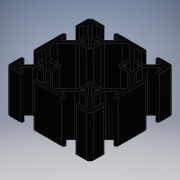
# Autodesk Inventor part: 2020-S-BLACK-FB
Saved by Autodesk Inventor 2017 SP1 (Build 210196100, 196)
## iProperties
Created: 2016-09-13
Part Number: 2020-S-BLACK-FB
Material: 6105-T5
Description: 40 S SHORT SINGLE UNIBEARING ASSEMBLY ON 40-4040 X 75mm
Document SubType Name: Modeling
Designer: BRALEF
Density: 1 g/cm^3
Appearance: BLACK ANODIZED
MATERIAL: 6061-T6
PART PRICE: 44.65
Author: BRALEF
Autodesk Inventor part; units mm, degrees
ref_plane "YZ Plane" through (0, 0, 0) normal (1, 0, 0) x (0, 1, 0)
ref_plane "XZ Plane" through (0, 0, 0) normal (0, 1, 0) x (-1, 0, 0)
ref_plane "XY Plane" through (0, 0, 0) normal (0, 0, 1) x (1, 0, 0)
sketch "Sketch1" plane through (0, 0, 0) normal (0, 1, 0) x (-1, 0, 0)
  arc A0 (-4.5172, 2.0392) -> (-5.1644, 3.6017) centre (-6.727, 2.0392) ccw
  line L0 (-10.6413, 9.0787) -> (-5.1644, 3.6017)
  arc A1 (-10.6413, 9.0787) -> (-14.7587, 9.0787) centre (-12.7, 7.02) ccw
  line L1 (-20.2356, 3.6017) -> (-14.7587, 9.0787)
  arc A2 (-20.2356, 3.6017) -> (-20.8828, 2.0392) centre (-18.673, 2.0392) ccw
  line L2 (-20.8828, -2.3074) -> (-20.8828, 2.0392)
  arc A3 (-23.0926, -4.5172) -> (-20.8828, -2.3074) centre (-23.0926, -2.3074) ccw
  line L3 (-27.4392, -4.5172) -> (-23.0926, -4.5172)
  arc A4 (-27.4392, -4.5172) -> (-29.0017, -5.1644) centre (-27.4392, -6.727) ccw
  line L4 (-34.4787, -10.6413) -> (-29.0017, -5.1644)
  arc A5 (-34.4787, -10.6413) -> (-34.4787, -14.7587) centre (-32.42, -12.7) ccw
  line L5 (-29.0017, -20.2356) -> (-34.4787, -14.7587)
  arc A6 (-29.0017, -20.2356) -> (-27.4392, -20.8828) centre (-27.4392, -18.673) ccw
  line L6 (-23.0926, -20.8828) -> (-27.4392, -20.8828)
  arc A7 (-20.8828, -23.0926) -> (-23.0926, -20.8828) centre (-23.0926, -23.0926) ccw
  line L7 (-20.8828, -27.4392) -> (-20.8828, -23.0926)
  arc A8 (-20.8828, -27.4392) -> (-20.2356, -29.0017) centre (-18.673, -27.4392) ccw
  line L8 (-14.7587, -34.4787) -> (-20.2356, -29.0017)
  arc A9 (-14.7587, -34.4787) -> (-10.6413, -34.4787) centre (-12.7, -32.42) ccw
  line L9 (-5.1644, -29.0017) -> (-10.6413, -34.4787)
  arc A10 (-5.1644, -29.0017) -> (-4.5172, -27.4392) centre (-6.727, -27.4392) ccw
  line L10 (-4.5172, -23.0926) -> (-4.5172, -27.4392)
  arc A11 (-2.3074, -20.8828) -> (-4.5172, -23.0926) centre (-2.3074, -23.0926) ccw
  line L11 (2.0392, -20.8828) -> (-2.3074, -20.8828)
  arc A12 (2.0392, -20.8828) -> (3.6017, -20.2356) centre (2.0392, -18.673) ccw
  line L12 (9.0787, -14.7587) -> (3.6017, -20.2356)
  arc A13 (9.0787, -14.7587) -> (9.0787, -10.6413) centre (7.02, -12.7) ccw
  line L13 (3.6017, -5.1644) -> (9.0787, -10.6413)
  arc A14 (3.6017, -5.1644) -> (2.0392, -4.5172) centre (2.0392, -6.727) ccw
  line L14 (-2.3074, -4.5172) -> (2.0392, -4.5172)
  arc A15 (-4.5172, -2.3074) -> (-2.3074, -4.5172) centre (-2.3074, -2.3074) ccw
  line L15 (-4.5172, 2.0392) -> (-4.5172, -2.3074)
  arc A16 (-2.8605, -1.9692) -> (-1.9692, -2.8605) centre (-2.4696, -2.4696) ccw
  line L16 (-1.3405, -2.2319) -> (-1.9692, -2.8605)
  arc A17 (-1.3405, -2.2319) -> (1.3405, -2.2319) centre (0, 0) ccw
  line L17 (1.9692, -2.8605) -> (1.3405, -2.2319)
  arc A18 (1.9692, -2.8605) -> (2.8605, -1.9692) centre (2.4696, -2.4696) ccw
  line L18 (2.2319, -1.3405) -> (2.8605, -1.9692)
  arc A19 (2.2319, -1.3405) -> (2.2319, 1.3405) centre (0, 0) ccw
  line L19 (2.8605, 1.9692) -> (2.2319, 1.3405)
  arc A20 (2.8605, 1.9692) -> (1.9692, 2.8605) centre (2.4696, 2.4696) ccw
  line L20 (1.3405, 2.2319) -> (1.9692, 2.8605)
  arc A21 (1.3405, 2.2319) -> (-1.3405, 2.2319) centre (0, 0) ccw
  line L21 (-1.9692, 2.8605) -> (-1.3405, 2.2319)
  arc A22 (-1.9692, 2.8605) -> (-2.8605, 1.9692) centre (-2.4696, 2.4696) ccw
  line L22 (-2.2319, 1.3405) -> (-2.8605, 1.9692)
  arc A23 (-2.2319, 1.3405) -> (-2.2319, -1.3405) centre (0, 0) ccw
  line L23 (-2.8605, -1.9692) -> (-2.2319, -1.3405)
  arc A24 (-28.2605, -1.9692) -> (-27.3692, -2.8605) centre (-27.8696, -2.4696) ccw
  line L24 (-26.7405, -2.2319) -> (-27.3692, -2.8605)
  arc A25 (-26.7405, -2.2319) -> (-24.0595, -2.2319) centre (-25.4, 0) ccw
  line L25 (-23.4308, -2.8605) -> (-24.0595, -2.2319)
  arc A26 (-23.4308, -2.8605) -> (-22.5395, -1.9692) centre (-22.9304, -2.4696) ccw
  line L26 (-23.1681, -1.3405) -> (-22.5395, -1.9692)
  arc A27 (-23.1681, -1.3405) -> (-23.1681, 1.3405) centre (-25.4, 0) ccw
  line L27 (-22.5395, 1.9692) -> (-23.1681, 1.3405)
  arc A28 (-22.5395, 1.9692) -> (-23.4308, 2.8605) centre (-22.9304, 2.4696) ccw
  line L28 (-24.0595, 2.2319) -> (-23.4308, 2.8605)
  arc A29 (-24.0595, 2.2319) -> (-26.7405, 2.2319) centre (-25.4, 0) ccw
  line L29 (-27.3692, 2.8605) -> (-26.7405, 2.2319)
  arc A30 (-27.3692, 2.8605) -> (-28.2605, 1.9692) centre (-27.8696, 2.4696) ccw
  line L30 (-27.6319, 1.3405) -> (-28.2605, 1.9692)
  arc A31 (-27.6319, 1.3405) -> (-27.6319, -1.3405) centre (-25.4, 0) ccw
  line L31 (-28.2605, -1.9692) -> (-27.6319, -1.3405)
  arc A32 (1.3405, -23.1681) -> (-1.3405, -23.1681) centre (0, -25.4) ccw
  line L32 (-1.9692, -22.5395) -> (-1.3405, -23.1681)
  arc A33 (-1.9692, -22.5395) -> (-2.8605, -23.4308) centre (-2.4696, -22.9304) ccw
  line L33 (-2.2319, -24.0595) -> (-2.8605, -23.4308)
  arc A34 (-2.2319, -24.0595) -> (-2.2319, -26.7405) centre (0, -25.4) ccw
  line L34 (-2.8605, -27.3692) -> (-2.2319, -26.7405)
  arc A35 (-2.8605, -27.3692) -> (-1.9692, -28.2605) centre (-2.4696, -27.8696) ccw
  line L35 (-1.3405, -27.6319) -> (-1.9692, -28.2605)
  arc A36 (-1.3405, -27.6319) -> (1.3405, -27.6319) centre (0, -25.4) ccw
  line L36 (1.9692, -28.2605) -> (1.3405, -27.6319)
  arc A37 (1.9692, -28.2605) -> (2.8605, -27.3692) centre (2.4696, -27.8696) ccw
  line L37 (2.2319, -26.7405) -> (2.8605, -27.3692)
  arc A38 (2.2319, -26.7405) -> (2.2319, -24.0595) centre (0, -25.4) ccw
  line L38 (2.8605, -23.4308) -> (2.2319, -24.0595)
  arc A39 (2.8605, -23.4308) -> (1.9692, -22.5395) centre (2.4696, -22.9304) ccw
  line L39 (1.3405, -23.1681) -> (1.9692, -22.5395)
  arc A40 (-28.2605, -27.3692) -> (-27.3692, -28.2605) centre (-27.8696, -27.8696) ccw
  line L40 (-26.7405, -27.6319) -> (-27.3692, -28.2605)
  arc A41 (-26.7405, -27.6319) -> (-24.0595, -27.6319) centre (-25.4, -25.4) ccw
  line L41 (-23.4308, -28.2605) -> (-24.0595, -27.6319)
  arc A42 (-23.4308, -28.2605) -> (-22.5395, -27.3692) centre (-22.9304, -27.8696) ccw
  line L42 (-23.1681, -26.7405) -> (-22.5395, -27.3692)
  arc A43 (-23.1681, -26.7405) -> (-23.1681, -24.0595) centre (-25.4, -25.4) ccw
  line L43 (-22.5395, -23.4308) -> (-23.1681, -24.0595)
  arc A44 (-22.5395, -23.4308) -> (-23.4308, -22.5395) centre (-22.9304, -22.9304) ccw
  line L44 (-24.0595, -23.1681) -> (-23.4308, -22.5395)
  arc A45 (-24.0595, -23.1681) -> (-26.7405, -23.1681) centre (-25.4, -25.4) ccw
  line L45 (-27.3692, -22.5395) -> (-26.7405, -23.1681)
  arc A46 (-27.3692, -22.5395) -> (-28.2605, -23.4308) centre (-27.8696, -22.9304) ccw
  line L46 (-27.6319, -24.0595) -> (-28.2605, -23.4308)
  arc A47 (-27.6319, -24.0595) -> (-27.6319, -26.7405) centre (-25.4, -25.4) ccw
  line L47 (-28.2605, -27.3692) -> (-27.6319, -26.7405)
  arc A48 (12.7, -29.7561) -> (10.4902, -29.7561) centre (11.5951, -29.7561) ccw
  line L48 (12.7, -29.7561) -> (12.7, -35.9918)
  arc A49 (10.5918, -38.1) -> (12.7, -35.9918) centre (10.5918, -35.9918) ccw
  line L49 (10.5918, -38.1) -> (4.3561, -38.1)
  arc A50 (4.3561, -35.8902) -> (4.3561, -38.1) centre (4.3561, -36.9951) ccw
  line L50 (4.3561, -35.8902) -> (6.4749, -35.8902)
  arc A51 (6.4749, -35.8902) -> (7.1933, -34.1558) centre (6.4749, -34.8742) ccw
  line L51 (7.1933, -34.1558) -> (3.8846, -30.8471)
  arc A52 (3.8846, -30.8471) -> (1.6396, -29.9172) centre (1.6396, -33.0922) ccw
  line L52 (1.6396, -29.9172) -> (-1.6396, -29.9172)
  arc A53 (-1.6396, -29.9172) -> (-3.8846, -30.8471) centre (-1.6396, -33.0922) ccw
  line L53 (-3.8846, -30.8471) -> (-7.1933, -34.1558)
  arc A54 (-7.1933, -34.1558) -> (-6.4749, -35.8902) centre (-6.4749, -34.8742) ccw
  line L54 (-6.4749, -35.8902) -> (-4.3561, -35.8902)
  arc A55 (-4.3561, -38.1) -> (-4.3561, -35.8902) centre (-4.3561, -36.9951) ccw
  line L55 (-4.3561, -38.1) -> (-21.0439, -38.1)
  arc A56 (-21.0439, -35.8902) -> (-21.0439, -38.1) centre (-21.0439, -36.9951) ccw
  line L56 (-21.0439, -35.8902) -> (-18.9251, -35.8902)
  arc A57 (-18.9251, -35.8902) -> (-18.2067, -34.1558) centre (-18.9251, -34.8742) ccw
  line L57 (-18.2067, -34.1558) -> (-21.5154, -30.8471)
  arc A58 (-21.5154, -30.8471) -> (-23.7604, -29.9172) centre (-23.7604, -33.0922) ccw
  line L58 (-23.7604, -29.9172) -> (-27.0396, -29.9172)
  arc A59 (-27.0396, -29.9172) -> (-29.2846, -30.8471) centre (-27.0396, -33.0922) ccw
  line L59 (-29.2846, -30.8471) -> (-32.5933, -34.1558)
  arc A60 (-32.5933, -34.1558) -> (-31.8749, -35.8902) centre (-31.8749, -34.8742) ccw
  line L60 (-31.8749, -35.8902) -> (-29.7561, -35.8902)
  arc A61 (-29.7561, -38.1) -> (-29.7561, -35.8902) centre (-29.7561, -36.9951) ccw
  line L61 (-29.7561, -38.1) -> (-35.9918, -38.1)
  arc A62 (-38.1, -35.9918) -> (-35.9918, -38.1) centre (-35.9918, -35.9918) ccw
  line L62 (-38.1, -35.9918) -> (-38.1, -29.7561)
  arc A63 (-35.8902, -29.7561) -> (-38.1, -29.7561) centre (-36.9951, -29.7561) ccw
  line L63 (-35.8902, -29.7561) -> (-35.8902, -31.8749)
  arc A64 (-35.8902, -31.8749) -> (-34.1558, -32.5933) centre (-34.8742, -31.8749) ccw
  line L64 (-34.1558, -32.5933) -> (-30.8471, -29.2846)
  arc A65 (-30.8471, -29.2846) -> (-29.9172, -27.0396) centre (-33.0922, -27.0396) ccw
  line L65 (-29.9172, -27.0396) -> (-29.9172, -23.7604)
  arc A66 (-29.9172, -23.7604) -> (-30.8471, -21.5154) centre (-33.0922, -23.7604) ccw
  line L66 (-30.8471, -21.5154) -> (-34.1558, -18.2067)
  arc A67 (-34.1558, -18.2067) -> (-35.8902, -18.9251) centre (-34.8742, -18.9251) ccw
  line L67 (-35.8902, -18.9251) -> (-35.8902, -21.0439)
  arc A68 (-38.1, -21.0439) -> (-35.8902, -21.0439) centre (-36.9951, -21.0439) ccw
  line L68 (-38.1, -21.0439) -> (-38.1, -4.3561)
  arc A69 (-35.8902, -4.3561) -> (-38.1, -4.3561) centre (-36.9951, -4.3561) ccw
  line L69 (-35.8902, -4.3561) -> (-35.8902, -6.4749)
  arc A70 (-35.8902, -6.4749) -> (-34.1558, -7.1933) centre (-34.8742, -6.4749) ccw
  line L70 (-34.1558, -7.1933) -> (-30.8471, -3.8846)
  arc A71 (-30.8471, -3.8846) -> (-29.9172, -1.6396) centre (-33.0922, -1.6396) ccw
  line L71 (-29.9172, -1.6396) -> (-29.9172, 1.6396)
  arc A72 (-29.9172, 1.6396) -> (-30.8471, 3.8846) centre (-33.0922, 1.6396) ccw
  line L72 (-30.8471, 3.8846) -> (-34.1558, 7.1933)
  arc A73 (-34.1558, 7.1933) -> (-35.8902, 6.4749) centre (-34.8742, 6.4749) ccw
  line L73 (-35.8902, 6.4749) -> (-35.8902, 4.3561)
  arc A74 (-38.1, 4.3561) -> (-35.8902, 4.3561) centre (-36.9951, 4.3561) ccw
  line L74 (-38.1, 4.3561) -> (-38.1, 10.5918)
  arc A75 (-35.9918, 12.7) -> (-38.1, 10.5918) centre (-35.9918, 10.5918) ccw
  line L75 (-35.9918, 12.7) -> (-29.7561, 12.7)
  arc A76 (-29.7561, 10.4902) -> (-29.7561, 12.7) centre (-29.7561, 11.5951) ccw
  line L76 (-29.7561, 10.4902) -> (-31.8749, 10.4902)
  arc A77 (-31.8749, 10.4902) -> (-32.5933, 8.7558) centre (-31.8749, 9.4742) ccw
  line L77 (-32.5933, 8.7558) -> (-29.2846, 5.4471)
  arc A78 (-29.2846, 5.4471) -> (-27.0396, 4.5172) centre (-27.0396, 7.6922) ccw
  line L78 (-27.0396, 4.5172) -> (-23.7604, 4.5172)
  arc A79 (-23.7604, 4.5172) -> (-21.5154, 5.4471) centre (-23.7604, 7.6922) ccw
  line L79 (-21.5154, 5.4471) -> (-18.2067, 8.7558)
  arc A80 (-18.2067, 8.7558) -> (-18.9251, 10.4902) centre (-18.9251, 9.4742) ccw
  line L80 (-18.9251, 10.4902) -> (-21.0439, 10.4902)
  arc A81 (-21.0439, 12.7) -> (-21.0439, 10.4902) centre (-21.0439, 11.5951) ccw
  line L81 (-21.0439, 12.7) -> (-4.3561, 12.7)
  arc A82 (-4.3561, 10.4902) -> (-4.3561, 12.7) centre (-4.3561, 11.5951) ccw
  line L82 (-4.3561, 10.4902) -> (-6.4749, 10.4902)
  arc A83 (-6.4749, 10.4902) -> (-7.1933, 8.7558) centre (-6.4749, 9.4742) ccw
  line L83 (-7.1933, 8.7558) -> (-3.8846, 5.4471)
  arc A84 (-3.8846, 5.4471) -> (-1.6396, 4.5172) centre (-1.6396, 7.6922) ccw
  line L84 (-1.6396, 4.5172) -> (1.6396, 4.5172)
  arc A85 (1.6396, 4.5172) -> (3.8846, 5.4471) centre (1.6396, 7.6922) ccw
  line L85 (3.8846, 5.4471) -> (7.1933, 8.7558)
  arc A86 (7.1933, 8.7558) -> (6.4749, 10.4902) centre (6.4749, 9.4742) ccw
  line L86 (6.4749, 10.4902) -> (4.3561, 10.4902)
  arc A87 (4.3561, 12.7) -> (4.3561, 10.4902) centre (4.3561, 11.5951) ccw
  line L87 (4.3561, 12.7) -> (10.5918, 12.7)
  arc A88 (12.7, 10.5918) -> (10.5918, 12.7) centre (10.5918, 10.5918) ccw
  line L88 (12.7, 10.5918) -> (12.7, 4.3561)
  arc A89 (10.4902, 4.3561) -> (12.7, 4.3561) centre (11.5951, 4.3561) ccw
  line L89 (10.4902, 4.3561) -> (10.4902, 6.4749)
  arc A90 (10.4902, 6.4749) -> (8.7558, 7.1933) centre (9.4742, 6.4749) ccw
  line L90 (8.7558, 7.1933) -> (5.4471, 3.8846)
  arc A91 (5.4471, 3.8846) -> (4.5172, 1.6396) centre (7.6922, 1.6396) ccw
  line L91 (4.5172, 1.6396) -> (4.5172, -1.6396)
  arc A92 (4.5172, -1.6396) -> (5.4471, -3.8846) centre (7.6922, -1.6396) ccw
  line L92 (5.4471, -3.8846) -> (8.7558, -7.1933)
  arc A93 (8.7558, -7.1933) -> (10.4902, -6.4749) centre (9.4742, -6.4749) ccw
  line L93 (10.4902, -6.4749) -> (10.4902, -4.3561)
  arc A94 (12.7, -4.3561) -> (10.4902, -4.3561) centre (11.5951, -4.3561) ccw
  line L94 (12.7, -4.3561) -> (12.7, -21.0439)
  arc A95 (10.4902, -21.0439) -> (12.7, -21.0439) centre (11.5951, -21.0439) ccw
  line L95 (10.4902, -21.0439) -> (10.4902, -18.9251)
  arc A96 (10.4902, -18.9251) -> (8.7558, -18.2067) centre (9.4742, -18.9251) ccw
  line L96 (8.7558, -18.2067) -> (5.4471, -21.5154)
  arc A97 (5.4471, -21.5154) -> (4.5172, -23.7604) centre (7.6922, -23.7604) ccw
  line L97 (4.5172, -23.7604) -> (4.5172, -27.0396)
  arc A98 (4.5172, -27.0396) -> (5.4471, -29.2846) centre (7.6922, -27.0396) ccw
  line L98 (5.4471, -29.2846) -> (8.7558, -32.5933)
  arc A99 (8.7558, -32.5933) -> (10.4902, -31.8749) centre (9.4742, -31.8749) ccw
  line L99 (10.4902, -31.8749) -> (10.4902, -29.7561)
  point P0 (0, 0)
  constraints: 200 end point, 200 point on circle, 136 tangent, 100 centre point, 68 equal radius, 36 parallel, 1 horizontal, 1 perpendicular, 1 vertical
extrude "Extrusion1" add sketch "Sketch1" along normal mid plane 25.4
body "Solid1"
